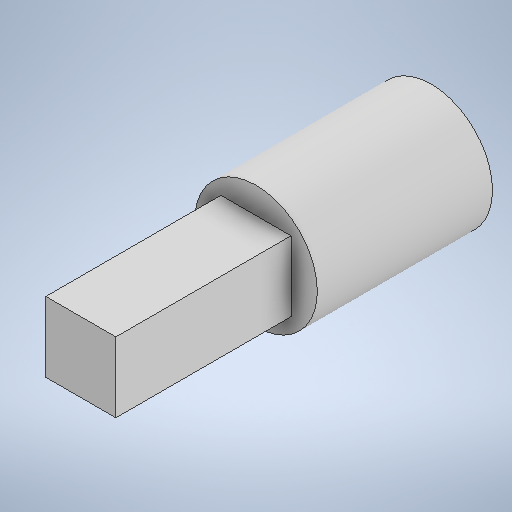
# Autodesk Inventor part: Geared Motor Transmission
Saved by Autodesk Inventor 2025.4 (Build 294407000, 407)
## iProperties
Created: 2026-05-09
Part Number: Geared Motor Transmission
Material: Generic
Document SubType Name: Modeling
Designer: lenovo
Density: 1 g/cm^3
Appearance: Default
Author: lenovo
Autodesk Inventor part; units mm, degrees
ref_plane "YZ Plane" through (0, 0, 0) normal (1, 0, 0) x (0, 1, 0)
ref_plane "XZ Plane" through (0, 0, 0) normal (0, 1, 0) x (-1, 0, 0)
ref_plane "XY Plane" through (0, 0, 0) normal (0, 0, 1) x (1, 0, 0)
sketch "Sketch1" plane through (0, 0, 0) normal (0, 0, 1) x (1, 0, 0)
  circle A0 centre (0, 0) radius 3.5
  line L0 (1.86, 1.9571) -> (1.86, -1.9571)
  line L1 (0, 3.5) -> (0, -3.5)
  line L2 (-1.86, 1.9571) -> (-1.86, -1.9571)
  arc A1 (-1.86, -1.9571) -> (1.86, -1.9571) centre (0, 0) ccw
  arc A2 (1.86, 1.9571) -> (-1.86, 1.9571) centre (0, 0) ccw
  dimension "d0" = 7
  dimension "d1" = 2.7
  dimension "d2" = 3.72
  constraints: 6 end point, 6 point on circle, 3 centre point, 3 coincident, 2 symmetric about line, 2 vertical, 1 concentric, 1 midpoint
  measures "d0" diameter of A0
  measures "d1" radius of A2
  measures "d2" diameter of L0 L1
extrude "Extrusion1" add sketch "Sketch1" along normal blind 7 contours A0 L1 A1 L0 A2 | L1 A2 L2 A1 A0
sketch "Sketch2" plane through (0, 0, 7) normal (0, 0, 1) x (1, 0, 0)
  circle A0 centre (0, 0) radius 3.5
  circle A1 centre (0, 0) radius 3.5 projected
  constraints: 1 centre point, 1 coincident, 1 concentric
extrude "Extrusion2" add sketch "Sketch2" along normal blind 3
sketch "Sketch3" plane through (0, 0, 10) normal (0, 0, 1) x (1, 0, 0)
  line L0 (-2, -2) -> (2, -2)
  line L1 (2, -2) -> (2, 2)
  line L2 (2, 2) -> (-2, 2)
  line L3 (-2, 2) -> (-2, -2)
  line L4 (-2, -2) -> (2, 2) construction
  line L5 (2, -2) -> (-2, 2) construction
  point P0 (0, 0)
  dimension "d7" = 4
  dimension "d8" = 4
  constraints: 12 end point, 2 midpoint, 2 parallel, 1 horizontal, 1 perpendicular
  measures "d7" distance of L2.end L1.end
  measures "d8" distance of L1.end L0.end
extrude "Extrusion3" add sketch "Sketch3" along normal blind 10
body "Solid1"
